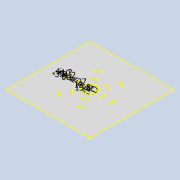
# Autodesk Inventor part: layer_1
Saved by Autodesk Inventor 2020 (Build 240168000, 168)
## iProperties
Created: 2021-10-03
Part Number: layer_1
Material: Generic
Document SubType Name: Modeling
Designer: Shuang Peng
Density: 1 g/cm^3
Appearance: Default
Author: Shuang Peng
Autodesk Inventor part; units mm, degrees
ref_plane "YZ Plane" through (0, 0, 0) normal (1, 0, 0) x (0, 1, 0)
ref_plane "XZ Plane" through (0, 0, 0) normal (0, 1, 0) x (-1, 0, 0)
ref_plane "XY Plane" through (0, 0, 0) normal (0, 0, 1) x (1, 0, 0)
sketch "Sketch1" plane through (0, 0, 0) normal (0, 1, 0) x (-1, 0, 0)
  line L0 (0, 0) -> (100, 0)
  line L1 (100, 0) -> (100, -100)
  line L2 (100, -100) -> (0, -100)
  line L3 (0, -100) -> (0, 0)
  dimension "d0" = 100
  dimension "d1" = 100
  constraints: 8 end point, 2 parallel, 1 horizontal, 1 perpendicular
  measures "d0" distance of L1.end L2.end
  measures "d1" distance of L0.end L1.end
extrude "Extrusion1" add sketch "Sketch1" along normal blind 0.3
sketch "Sketch2" plane through (0, 0.3, 0) normal (0, 1, 0) x (1, 0, 0)
  line L0 (-100, 100) -> (-100, 0) projected
  line L1 (-100, 0) -> (0, 0) projected
  line L2 (0, 0) -> (0, 100) projected
  line L3 (0, 100) -> (-100, 100) projected
  line L4 (0, 0) -> (0, 50)
  line L5 (0, 0) -> (0, 100) projected
  line L6 (0, 50) -> (-50, 50)
  circle A0 centre (-50, 50) radius 1.5
  dimension "d4" = 50
  dimension "d5" = 3
  constraints: 4 end point, 1 centre point, 1 coincident, 1 midpoint, 1 perpendicular
  measures "d4" distance of L4.end L6.end
  measures "d5" diameter of A0
extrude "Extrusion2" cut sketch "Sketch2" against normal blind 0.3 contours A0
sketch "Sketch3" plane through (0, 0.3, 0) normal (0, 1, 0) x (1, 0, 0)
  circle A0 centre (-50, 50) radius 1.5 projected
  line L0 (-100, 100) -> (-100, 0) projected
  line L1 (-100, 0) -> (0, 0) projected
  line L2 (0, 0) -> (0, 100) projected
  line L3 (0, 100) -> (-100, 100) projected
  line L4 (-50, 50) -> (-57, 50)
  line L5 (-57, 47.5) -> (-57, 52.5) construction
  line L6 (-56.9, 47.5) -> (-56.9, 52.5)
  line L7 (-57.1, 52.5) -> (-57.1, 47.5)
  arc A1 (-57.1, 47.5) -> (-56.9, 47.5) centre (-57, 47.5) ccw
  arc A2 (-56.9, 52.5) -> (-57.1, 52.5) centre (-57, 52.5) ccw
  line L8 (-57, 50) -> (-65, 50)
  line L9 (-65, 47.5) -> (-65, 52.5) construction
  line L10 (-64.9, 47.5) -> (-64.9, 52.5)
  line L11 (-65.1, 52.5) -> (-65.1, 47.5)
  arc A3 (-65.1, 47.5) -> (-64.9, 47.5) centre (-65, 47.5) ccw
  arc A4 (-64.9, 52.5) -> (-65.1, 52.5) centre (-65, 52.5) ccw
  line L12 (-65, 50) -> (-77, 50)
  line L13 (-77, 47.5) -> (-77, 52.5) construction
  line L14 (-76.9, 47.5) -> (-76.9, 52.5)
  line L15 (-77.1, 52.5) -> (-77.1, 47.5)
  arc A5 (-77.1, 47.5) -> (-76.9, 47.5) centre (-77, 47.5) ccw
  arc A6 (-76.9, 52.5) -> (-77.1, 52.5) centre (-77, 52.5) ccw
  dimension "d8" = 7
  dimension "d9" = 2.5
  dimension "d10" = 0.2
  dimension "d11" = 8
  dimension "d12" = 2.5
  dimension "d13" = 0.2
  dimension "d14" = 12
  dimension "d15" = 2.5
  dimension "d16" = 0.2
  constraints: 30 end point, 12 point on circle, 12 tangent, 6 centre point, 3 horizontal, 3 midpoint, 3 parallel, 3 vertical
  measures "d8" distance of L4.start L4.end
  measures "d9" distance of L4.end L5.end
  measures "d10" diameter of A2
  measures "d11" distance of L4.end L8.end
  measures "d12" distance of L8.end L9.end
  measures "d13" diameter of A4
  measures "d14" distance of L8.end L12.end
  measures "d15" distance of L12.end L13.end
  measures "d16" diameter of A6
extrude "Extrusion3" cut sketch "Sketch3" against normal blind 0.3 contours L14 A5 L15 A6 | L10 A3 L11 L12 L8 | L8 L12 L11 A4 L10 | L6 A1 L7 L8 L4 | L4 L8 L7 A2 L6
pattern_circular "Circular Pattern1" count 6 over 360 about axis through (-50, 0.3, -50) along (0, -1, 0) of "Extrusion3"
sketch "Sketch4" plane through (0, 0.3, 0) normal (0, 1, 0) x (1, 0, 0)
  line L0 (-51.3849, 42.6012) -> (-55.7151, 45.1012) projected
  arc A0 (-55.6151, 45.2744) -> (-55.7151, 45.1012) centre (-55.6651, 45.1878) ccw projected
  line L1 (-55.6151, 45.2744) -> (-51.2849, 42.7744) projected
  arc A1 (-51.3849, 42.6012) -> (-51.2849, 42.7744) centre (-51.3349, 42.6878) ccw projected
  line L2 (-55.3849, 35.673) -> (-59.7151, 38.173) projected
  arc A2 (-59.6151, 38.3462) -> (-59.7151, 38.173) centre (-59.6651, 38.2596) ccw projected
  line L3 (-59.6151, 38.3462) -> (-55.2849, 35.8462) projected
  arc A3 (-55.3849, 35.673) -> (-55.2849, 35.8462) centre (-55.3349, 35.7596) ccw projected
  arc A4 (-65.6151, 27.9539) -> (-65.7151, 27.7807) centre (-65.6651, 27.8673) ccw projected
  line L4 (-65.6151, 27.9539) -> (-61.2849, 25.4539) projected
  arc A5 (-61.3849, 25.2807) -> (-61.2849, 25.4539) centre (-61.3349, 25.3673) ccw projected
  line L5 (-61.3849, 25.2807) -> (-65.7151, 27.7807) projected
  line L6 (-44.2849, 45.1012) -> (-48.6151, 42.6012) projected
  arc A6 (-48.7151, 42.7744) -> (-48.6151, 42.6012) centre (-48.6651, 42.6878) ccw projected
  line L7 (-48.7151, 42.7744) -> (-44.3849, 45.2744) projected
  arc A7 (-44.2849, 45.1012) -> (-44.3849, 45.2744) centre (-44.3349, 45.1878) ccw projected
  line L8 (-40.2849, 38.173) -> (-44.6151, 35.673) projected
  arc A8 (-44.7151, 35.8462) -> (-44.6151, 35.673) centre (-44.6651, 35.7596) ccw projected
  line L9 (-44.7151, 35.8462) -> (-40.3849, 38.3462) projected
  arc A9 (-40.2849, 38.173) -> (-40.3849, 38.3462) centre (-40.3349, 38.2596) ccw projected
  arc A10 (-38.7151, 25.4539) -> (-38.6151, 25.2807) centre (-38.6651, 25.3673) ccw projected
  line L10 (-38.7151, 25.4539) -> (-34.3849, 27.9539) projected
  arc A11 (-34.2849, 27.7807) -> (-34.3849, 27.9539) centre (-34.3349, 27.8673) ccw projected
  line L11 (-34.2849, 27.7807) -> (-38.6151, 25.2807) projected
  line L12 (-42.9, 52.5) -> (-42.9, 47.5) projected
  arc A12 (-43.1, 47.5) -> (-42.9, 47.5) centre (-43, 47.5) ccw projected
  line L13 (-43.1, 47.5) -> (-43.1, 52.5) projected
  arc A13 (-42.9, 52.5) -> (-43.1, 52.5) centre (-43, 52.5) ccw projected
  line L14 (-34.9, 52.5) -> (-34.9, 47.5) projected
  arc A14 (-35.1, 47.5) -> (-34.9, 47.5) centre (-35, 47.5) ccw projected
  line L15 (-35.1, 47.5) -> (-35.1, 52.5) projected
  arc A15 (-34.9, 52.5) -> (-35.1, 52.5) centre (-35, 52.5) ccw projected
  arc A16 (-23.1, 47.5) -> (-22.9, 47.5) centre (-23, 47.5) ccw projected
  line L16 (-23.1, 47.5) -> (-23.1, 52.5) projected
  arc A17 (-22.9, 52.5) -> (-23.1, 52.5) centre (-23, 52.5) ccw projected
  line L17 (-22.9, 52.5) -> (-22.9, 47.5) projected
  line L18 (-48.6151, 57.3988) -> (-44.2849, 54.8988) projected
  arc A18 (-44.3849, 54.7256) -> (-44.2849, 54.8988) centre (-44.3349, 54.8122) ccw projected
  line L19 (-44.3849, 54.7256) -> (-48.7151, 57.2256) projected
  arc A19 (-48.6151, 57.3988) -> (-48.7151, 57.2256) centre (-48.6651, 57.3122) ccw projected
  line L20 (-44.6151, 64.327) -> (-40.2849, 61.827) projected
  arc A20 (-40.3849, 61.6538) -> (-40.2849, 61.827) centre (-40.3349, 61.7404) ccw projected
  line L21 (-40.3849, 61.6538) -> (-44.7151, 64.1538) projected
  arc A21 (-44.6151, 64.327) -> (-44.7151, 64.1538) centre (-44.6651, 64.2404) ccw projected
  arc A22 (-34.3849, 72.0461) -> (-34.2849, 72.2193) centre (-34.3349, 72.1327) ccw projected
  line L22 (-34.3849, 72.0461) -> (-38.7151, 74.5461) projected
  arc A23 (-38.6151, 74.7193) -> (-38.7151, 74.5461) centre (-38.6651, 74.6327) ccw projected
  line L23 (-38.6151, 74.7193) -> (-34.2849, 72.2193) projected
  line L24 (-55.7151, 54.8988) -> (-51.3849, 57.3988) projected
  arc A24 (-51.2849, 57.2256) -> (-51.3849, 57.3988) centre (-51.3349, 57.3122) ccw projected
  line L25 (-51.2849, 57.2256) -> (-55.6151, 54.7256) projected
  arc A25 (-55.7151, 54.8988) -> (-55.6151, 54.7256) centre (-55.6651, 54.8122) ccw projected
  line L26 (-59.7151, 61.827) -> (-55.3849, 64.327) projected
  arc A26 (-55.2849, 64.1538) -> (-55.3849, 64.327) centre (-55.3349, 64.2404) ccw projected
  line L27 (-55.2849, 64.1538) -> (-59.6151, 61.6538) projected
  arc A27 (-59.7151, 61.827) -> (-59.6151, 61.6538) centre (-59.6651, 61.7404) ccw projected
  arc A28 (-61.2849, 74.5461) -> (-61.3849, 74.7193) centre (-61.3349, 74.6327) ccw projected
  line L28 (-61.2849, 74.5461) -> (-65.6151, 72.0461) projected
  arc A29 (-65.7151, 72.2193) -> (-65.6151, 72.0461) centre (-65.6651, 72.1327) ccw projected
  line L29 (-65.7151, 72.2193) -> (-61.3849, 74.7193) projected
  line L30 (-57.1, 47.5) -> (-57.1, 52.5) projected
  arc A30 (-56.9, 52.5) -> (-57.1, 52.5) centre (-57, 52.5) ccw projected
  line L31 (-56.9, 52.5) -> (-56.9, 47.5) projected
  arc A31 (-57.1, 47.5) -> (-56.9, 47.5) centre (-57, 47.5) ccw projected
  line L32 (-65.1, 47.5) -> (-65.1, 52.5) projected
  arc A32 (-64.9, 52.5) -> (-65.1, 52.5) centre (-65, 52.5) ccw projected
  line L33 (-64.9, 52.5) -> (-64.9, 47.5) projected
  arc A33 (-65.1, 47.5) -> (-64.9, 47.5) centre (-65, 47.5) ccw projected
  arc A34 (-76.9, 52.5) -> (-77.1, 52.5) centre (-77, 52.5) ccw projected
  line L34 (-76.9, 52.5) -> (-76.9, 47.5) projected
  arc A35 (-77.1, 47.5) -> (-76.9, 47.5) centre (-77, 47.5) ccw projected
  line L35 (-77.1, 47.5) -> (-77.1, 52.5) projected
  circle A36 centre (-50, 50) radius 1.5 projected
  line L36 (0, 0) -> (0, 100) projected
  line L37 (0, 100) -> (-100, 100) projected
  line L38 (-100, 100) -> (-100, 0) projected
  line L39 (-100, 0) -> (0, 0) projected
  line L40 (-76.9, 47.5) -> (-76.9, 52.5) projected
  line L41 (-76.9, 50) -> (-77, 50)
  line L42 (-76.9, 52.5) -> (-76.9, 47.5) projected
  line L43 (-77, 50) -> (-82, 50)
  line L44 (-87, 48) -> (-87, 52)
  line L45 (-87, 52) -> (-77, 52)
  line L46 (-77, 52) -> (-77, 48)
  line L47 (-77, 48) -> (-87, 48)
  line L48 (-87, 48) -> (-77, 52) construction
  line L49 (-87, 52) -> (-77, 48) construction
  circle A37 centre (-82, 50) radius 0.6
  line L50 (-82, 50) -> (-85.5, 50)
  circle A38 centre (-85.5, 50) radius 0.6
  circle A39 centre (-50, 50) radius 1.5 projected
  line L51 (-50, 50) -> (-77, 50)
  circle A40 centre (-50, 50) radius 6
  line L52 (-50, 50) -> (-63.5, 50)
  line L53 (-50, 48) -> (-50, 52)
  line L54 (-50, 52) -> (-77, 52)
  line L55 (-77, 52) -> (-77, 48)
  line L56 (-77, 48) -> (-50, 48)
  line L57 (-50, 48) -> (-77, 52) construction
  line L58 (-50, 52) -> (-77, 48) construction
  dimension "d22" = 0.1
  dimension "d23" = 5
  dimension "d24" = 4
  dimension "d25" = 10
  dimension "d26" = 1.2
  dimension "d27" = 3.5
  dimension "d28" = 1.2
  dimension "d29" = 12
  dimension "d30" = 13.5
  dimension "d31" = 4
  dimension "d32" = 27
  constraints: 34 end point, 7 perpendicular, 6 midpoint, 4 parallel, 3 centre point, 3 coincident, 1 horizontal
  measures "d22" distance of L41.start L41.end
  measures "d23" distance of L41.end L43.end
  measures "d24" distance of L44.start L44.end
  measures "d25" distance of L44.end L45.end
  measures "d26" diameter of A37
  measures "d27" distance of L50.start L50.end
  measures "d28" diameter of A38
  measures "d29" diameter of A40
  measures "d30" distance of L52.start L52.end
  measures "d31" distance of L53.start L53.end
  measures "d32" distance of L54.end L53.end
body "Solid1"
